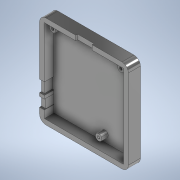
# Autodesk Inventor part: Base
Saved by Autodesk Inventor 2021 (Build 250183000, 183)
## iProperties
Created: 2020-12-21
Part Number: Base
Material: Generic
Document SubType Name: Modeling
Designer: Vitor
Density: 1 g/cm^3
Appearance: Default
Author: Vitor
Autodesk Inventor part; units mm, degrees
ref_plane "YZ Plane" through (0, 0, 0) normal (1, 0, 0) x (0, 1, 0)
ref_plane "XZ Plane" through (0, 0, 0) normal (0, 1, 0) x (-1, 0, 0)
sketch "Sketch1" plane through (0, 0, 0) normal (0, 0, 1) x (1, 0, 0)
  line L0 (0, 103.81) -> (0, 0)
  line L1 (99.04, 103.81) -> (0, 103.81)
  line L2 (99.04, 0) -> (99.04, 103.81)
  circle A0 centre (91.5302, 97.8155) radius 1.6
  circle A1 centre (6.3166, 98.2023) radius 1.6
  circle A2 centre (63.7434, 9.4559) radius 1.6
  line L3 (-2.8877, 39.67) -> (-2.8877, 25.07)
  line L4 (18.04, 39.67) -> (-2.8877, 39.67)
  line L5 (-2.8877, 25.07) -> (18.04, 25.07)
  line L6 (5.99, 20.97) -> (-0.5, 20.97)
  line L7 (-0.5, 20.97) -> (-0.5, 9.286)
  line L8 (-0.5, 9.286) -> (5.99, 9.286)
  line L9 (5.99, 9.286) -> (5.99, 20.97)
  line L10 (18.04, 25.07) -> (18.04, 39.67)
  line L11 (0, 0) -> (99.04, 0)
  line L12 (-2, 105.81) -> (-2, -2)
  line L13 (-2, -2) -> (101.04, -2)
  line L14 (101.04, -2) -> (101.04, 105.81)
  line L15 (101.04, 105.81) -> (-2, 105.81)
  line L16 (-6, 109.81) -> (-6, -6)
  line L17 (-6, -6) -> (105.04, -6)
  line L18 (105.04, -6) -> (105.04, 109.81)
  line L19 (105.04, 109.81) -> (-6, 109.81)
  point P0 (-2, 25.07)
  point P1 (-2, 39.67)
  point P2 (0, 39.67)
  point P3 (0, 9.286)
  point P4 (0, 20.97)
  point P5 (0, 25.07)
  dimension "d0" = 2
  dimension "d1" = 4
  constraints: 40 end point, 3 centre point, 2 horizontal, 2 vertical, 6 other
  measures "d0" distance between parallel lines of L1 L15
  measures "d1" distance between parallel lines of L15 L19
extrude "Extrusion1" add sketch "Sketch1" along normal blind 15 contours L0 L4 L12 L15 L14 L13 L5 L6 L7 L8 L11 L2 L1 | L12 L5 L3 L4 | L19 L18 L17 L16
extrude "Extrusion2" add sketch "Sketch1" along normal blind 3 contours L1 L2 L11 L0 L8 L9 L6 L5 L10 L4 | L4 L10 L5 L0 | L0 L5 L12 L4 | L6 L9 L8 L0 | L0 L8 L7 L6 | A0 | A1 | A2
sketch "Sketch2" plane through (0, 0, 3) normal (0, 0, 1) x (1, 0, 0)
  circle A0 centre (63.7434, 9.4559) radius 1.6 projected
  circle A1 centre (91.5302, 97.8155) radius 1.6 projected
  circle A2 centre (6.3166, 98.2023) radius 1.6 projected
  circle A3 centre (6.3166, 98.2023) radius 4
  circle A4 centre (91.5302, 97.8155) radius 4
  circle A5 centre (63.7434, 9.4559) radius 4
  point P0 (0, 0)
  dimension "d8" = 8
  dimension "d9" = 8
  dimension "d10" = 8
  constraints: 3 centre point, 3 coincident
  measures "d8" diameter of A3
  measures "d9" diameter of A4
  measures "d10" diameter of A5
extrude "Extrusion4" add sketch "Sketch2" along normal blind 8
ref_plane "Work Plane1" through (0, 0, 12.662) normal (0, 0, -1) x (-1, 0, 0)
sketch "Sketch3" plane through (0, 0, 12.662) normal (0, 0, -1) x (-1, 0, 0)
  line L0 (2, 25.07) -> (2, 39.67) projected
  line L1 (2, 39.67) -> (6, 39.67)
  line L2 (6, 109.81) -> (6, -6) projected
  line L3 (0, 20.97) -> (0, 25.07) projected
  line L4 (6, 39.67) -> (0, 39.67)
  line L5 (0, 39.67) -> (0, 25.07)
  line L6 (0, 25.07) -> (6, 25.07)
  line L7 (6, 25.07) -> (6, 39.67)
  line L8 (0.5, 20.97) -> (0, 20.97) projected
  line L9 (0.5, 20.97) -> (6, 20.97)
  line L10 (0, 9.286) -> (0.5, 9.286) projected
  line L11 (0.5, 9.286) -> (6, 9.286)
  line L12 (6, 9.286) -> (6, 20.97)
  line L13 (0.5, 9.286) -> (0.5, 20.97) projected
  line L14 (0.5, 20.97) -> (0.5, 9.286)
  point P0 (0, 0)
  constraints: 18 end point, 4 perpendicular, 3 point on line, 2 horizontal, 2 parallel, 1 vertical
extrude "Extrusion5" cut sketch "Sketch3" against normal blind 8 contours L6 L5 L4 L0 | L0 L1 L2 L6 | L2 L11 L13 L9
fillet "Fillet1" radius 8 4 edges at (-6, 109.81, 7.5) (-6, -6, 7.5) (105.04, -6, 7.5) (105.04, 109.81, 7.5)
sketch "Sketch4" plane through (0, 0, 15) normal (0, 0, 1) x (1, 0, 0)
  line L0 (97.04, 109.81) -> (2, 109.81) projected
  line L1 (2, 109.81) -> (97.04, 109.81)
  line L2 (0, 103.81) -> (99.04, 103.81) projected
  line L3 (39.4018, 103.81) -> (59.6382, 103.81)
  line L4 (59.6382, 103.81) -> (59.6382, 109.81)
  line L5 (59.6382, 109.81) -> (39.4018, 109.81)
  line L6 (39.4018, 109.81) -> (39.4018, 103.81)
  line L7 (39.4018, 103.81) -> (59.6382, 109.81) construction
  line L8 (59.6382, 103.81) -> (39.4018, 109.81) construction
  point P0 (0, 0)
  point P1 (49.52, 106.81)
  constraints: 14 end point, 2 horizontal, 2 midpoint, 2 parallel, 1 perpendicular, 1 point on line
extrude "Extrusion6" cut sketch "Sketch4" against normal up to surface (2.338 mm away)
body "Solid1"
